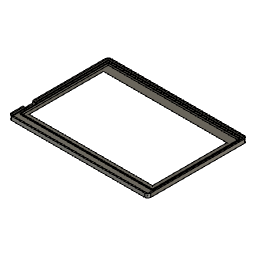
Soldered Inkplate 7 v1.0.0. Top v1.0.0. (Autodesk Fusion 360 design; units mm, degrees)
Autodesk Fusion 360 part; units mm, degrees
sketch "Sketch1" plane through (0, 0, 0) normal (0, 0, 1) x (1, 0, 0)
  line L0 (88.6, 66.25) -> (-88.6, 66.25)
  line L1 (-92.6, 62.25) -> (-92.6, -62.25)
  line L2 (-88.6, -66.25) -> (88.6, -66.25)
  line L3 (92.6, -62.25) -> (92.6, 62.25)
  line L4 (92.6, 66.25) -> (-92.6, -66.25) construction
  line L5 (-92.6, 66.25) -> (92.6, -66.25) construction
  line L6 (82.1, 49.46) -> (-82.1, 49.46)
  line L7 (-82.1, 49.46) -> (-82.1, -49.46)
  line L8 (-82.1, -49.46) -> (82.1, -49.46)
  line L9 (82.1, -49.46) -> (82.1, 49.46)
  line L10 (82.1, 49.46) -> (-82.1, -49.46) construction
  line L11 (-82.1, 49.46) -> (82.1, -49.46) construction
  arc A0 (-88.6, 66.25) -> (-92.6, 62.25) centre (-88.6, 62.25) ccw
  arc A1 (-92.6, -62.25) -> (-88.6, -66.25) centre (-88.6, -62.25) ccw
  arc A2 (88.6, -66.25) -> (92.6, -62.25) centre (88.6, -62.25) ccw
  arc A3 (92.6, 62.25) -> (88.6, 66.25) centre (88.6, 62.25) ccw
  dimension "d1" = 185.2
  dimension "d2" = 132.5
  dimension "d3" = 98.92
  dimension "d4" = 164.2
  dimension "d9" = 4
  constraint horizontal L0
  constraint perpendicular L0 L1
  constraint parallel L0 L2
  constraint parallel L1 L3
  constraint coincident L4 origin
  constraint coincident L5 origin
  constraint horizontal L6
  constraint perpendicular L6 L7
  constraint parallel L6 L8
  constraint parallel L7 L9
  constraint coincident L10 origin
  constraint coincident L11 origin
  constraint coincident L5.start L0
  constraint coincident L5.start L1
  constraint tangent L0 A0
  constraint tangent L1 A0
  constraint coincident L4.end L2
  constraint coincident L4.end L1
  constraint tangent L2 A1
  constraint tangent L1 A1
  constraint equal A0 A1
  constraint coincident L5.end L3
  constraint coincident L5.end L2
  constraint tangent L3 A2
  constraint tangent L2 A2
  constraint equal A0 A2
  constraint coincident L4.start L0
  constraint coincident L4.start L3
  constraint tangent L0 A3
  constraint tangent L3 A3
  constraint equal A0 A3
  measures "d1" distance of L4.end L5.end
  measures "d2" distance of L5.start L4.end
  measures "d3" distance of L6.end L7.end
  measures "d4" distance of L6.start L6.end
  measures "d9" radius of A0
extrude "Extrude1" add sketch "Sketch1" along normal blind 5
sketch "Sketch2" plane through (0, 0, 5) normal (0, 0, 1) x (-1, 0, 0)
  line L0 (-82.1, -49.46) -> (-82.1, 49.46)
  line L1 (-82.1, 49.46) -> (82.1, 49.46)
  line L2 (82.1, 49.46) -> (82.1, -49.46)
  line L3 (82.1, -49.46) -> (-82.1, -49.46)
  line L4 (-92.6, 62.25) -> (-92.6, -62.25)
  line L5 (-88.6, -66.25) -> (88.6, -66.25)
  line L6 (92.6, -62.25) -> (92.6, 62.25)
  line L7 (88.6, 66.25) -> (-88.6, 66.25)
  line L8 (-91.1, -64.75) -> (91.1, -64.75)
  line L9 (91.1, -64.75) -> (91.1, 64.75)
  line L10 (91.1, 64.75) -> (-91.1, 64.75)
  line L11 (-91.1, 64.75) -> (-91.1, -64.75)
  line L12 (-91.1, -64.75) -> (91.1, 64.75) construction
  line L13 (91.1, -64.75) -> (-91.1, 64.75) construction
  arc A0 (-92.6, -62.25) -> (-88.6, -66.25) centre (-88.6, -62.25) ccw
  arc A1 (88.6, -66.25) -> (92.6, -62.25) centre (88.6, -62.25) ccw
  arc A2 (92.6, 62.25) -> (88.6, 66.25) centre (88.6, 62.25) ccw
  arc A3 (-88.6, 66.25) -> (-92.6, 62.25) centre (-88.6, 62.25) ccw
  dimension "d7" = 1.5
  dimension "d8" = 1.5
  constraint horizontal L8
  constraint perpendicular L8 L9
  constraint parallel L8 L10
  constraint parallel L9 L11
  constraint coincident L12 origin
  constraint coincident L13 origin
  measures "d7" distance of L5 L8
  measures "d8" distance of L4 L11
extrude "Extrude2" cut sketch "Sketch2" against normal blind 3.1 contours L8 L9 L10 L11
chamfer "Chamfer1" distance 1.9 angle 45 4 edges at (-82.1, 0, 0) (0, -49.46, 0) (0, 49.46, 0) (82.1, 0, 0)
sketch "Sketch3" plane through (0, 0, 1.9) normal (0, 0, 1) x (-1, 0, 0)
  line L0 (82.1, 49.46) -> (82.1, -49.46)
  line L1 (82.1, -49.46) -> (-82.1, -49.46)
  line L2 (-82.1, -49.46) -> (-82.1, 49.46)
  line L3 (-82.1, 49.46) -> (82.1, 49.46)
  line L4 (-91.1, 64.75) -> (-91.1, -64.75)
  line L5 (-91.1, -64.75) -> (91.1, -64.75)
  line L6 (91.1, -64.75) -> (91.1, 64.75)
  line L7 (91.1, 64.75) -> (-91.1, 64.75)
  line L8 (0, 0) -> (0, -20) construction
  line L9 (-88.1, -61.75) -> (88.1, -61.75)
  line L10 (88.1, -61.75) -> (88.1, 55.45)
  line L11 (88.1, 55.45) -> (-88.1, 55.45)
  line L12 (-88.1, 55.45) -> (-88.1, -61.75)
  line L13 (-88.1, -61.75) -> (88.1, 55.45) construction
  line L14 (88.1, -61.75) -> (-88.1, 55.45) construction
  line L15 (-86.1, -59.75) -> (86.1, -59.75)
  line L16 (86.1, -59.75) -> (86.1, 53.45)
  line L17 (86.1, 53.45) -> (-86.1, 53.45)
  line L18 (-86.1, 53.45) -> (-86.1, -59.75)
  line L19 (-86.1, -59.75) -> (86.1, 53.45) construction
  line L20 (86.1, -59.75) -> (-86.1, 53.45) construction
  point P0 (0, -3.15)
  point P1 (0, -3.15)
  point P2 (0, -3.15)
  dimension "d19" = 3.15
  dimension "d20" = 3
  dimension "d21" = 3
  dimension "d22" = 2
  dimension "d23" = 2
  constraint coincident L8.start origin
  constraint vertical L8
  constraint coincident P2 L8
  constraint horizontal L9
  constraint perpendicular L9 L10
  constraint parallel L9 L11
  constraint parallel L10 L12
  constraint coincident L13 P2
  constraint coincident L14 P2
  constraint coincident P2 P1
  constraint horizontal L15
  constraint perpendicular L15 L16
  constraint parallel L15 L17
  constraint parallel L16 L18
  constraint coincident L19 P2
  constraint coincident L20 P2
  measures "d19" distance of L8.start P2
  measures "d20" distance of L5 L9
  measures "d21" distance of L4 L12
  measures "d22" distance of L9 L15
  measures "d23" distance of L12 L18
extrude "Extrude3" add sketch "Sketch3" along normal blind 1.2 contours L9 L10 L11 L12
chamfer "Chamfer2" distance 1.2 angle 45 4 edges at (0, 59.75, 3.1) (-86.1, 3.15, 3.1) (86.1, 3.15, 3.1) (0, -53.45, 3.1)
sketch "Sketch4" plane through (0, 0, 1.9) normal (0, 0, 1) x (-1, 0, 0)
  line L0 (-91.1, 64.75) -> (-91.1, -64.75)
  line L1 (-91.1, -64.75) -> (91.1, -64.75)
  line L2 (91.1, -64.75) -> (91.1, 64.75)
  line L3 (91.1, 64.75) -> (-91.1, 64.75)
  line L4 (-88.1, 55.45) -> (88.1, 55.45)
  line L5 (88.1, 55.45) -> (88.1, -61.75)
  line L6 (88.1, -61.75) -> (-88.1, -61.75)
  line L7 (-88.1, -61.75) -> (-88.1, 55.45)
  line L8 (88.1, 31.95) -> (91.1, 31.95)
  line L9 (91.1, 31.95) -> (91.1, 33.95)
  line L10 (91.1, 33.95) -> (88.1, 33.95)
  line L11 (88.1, 33.95) -> (88.1, 31.95)
  line L12 (89.1, 38.9967) -> (89.1, 53.7443) construction
  line L13 (92.6, -62.25) -> (92.6, 62.25)
  line L14 (89.1, 46.95) -> (88.1, 46.95)
  line L15 (88.1, 46.95) -> (88.1, 48.95)
  line L16 (88.1, 48.95) -> (89.1, 48.95)
  line L17 (89.1, 48.95) -> (89.1, 46.95)
  line L18 (88.6, 66.25) -> (-88.6, 66.25)
  dimension "d27" = 3.5
  dimension "d28" = 2
  dimension "d30" = 13
  dimension "d31" = 2
  dimension "d37" = 19.3
  constraint horizontal L8
  constraint vertical L9
  constraint horizontal L10
  constraint vertical L11
  constraint coincident L2 L9.end
  constraint coincident L5 L8.start
  constraint vertical L12
  constraint horizontal L14
  constraint vertical L15
  constraint horizontal L16
  constraint vertical L17
  constraint coincident L5 L15.end
  constraint coincident L12 L14.start
  measures "d27" distance of L12 L13
  measures "d28" distance of L14.start L16.end
  measures "d30" distance of L10 L14.start
  measures "d31" distance of L8.end L9.end
  measures "d37" vertical distance of L14.start L18.start
extrude "Extrude4" add sketch "Sketch4" along normal blind 3.1 contours L2 L5 L8 L9 L10 L11 | L5 L14 L15 L16 L17
sketch "Sketch5" plane through (-92.6, 0, 0) normal (-1, 0, 0) x (0, -1, 0)
  line L0 (-62.25, 0) -> (62.25, 0)
  line L1 (62.25, 0) -> (62.25, 5)
  line L2 (62.25, 5) -> (-62.25, 5)
  line L3 (-62.25, 5) -> (-62.25, 0)
  line L4 (46.95, 5) -> (33.95, 5)
  line L5 (33.95, 5) -> (33.95, 2)
  line L6 (33.95, 2) -> (46.95, 2)
  line L7 (46.95, 2) -> (46.95, 5)
  point P0 (66.25, 5)
  dimension "d34" = 13
  dimension "d35" = 3
  dimension "d36" = 19.3
  constraint horizontal L4
  constraint vertical L5
  constraint horizontal L6
  constraint vertical L7
  constraint coincident L2 L4.start
  measures "d34" distance of L4.start L4.end
  measures "d35" distance of L4.start L6.end
  measures "d36" distance of L4.start P0
extrude "Extrude5" cut sketch "Sketch5" against normal blind 2 contours L2 L4 L5 L6 L7
fillet "Fillet1" radius 2 4 edges at (-88.6, -46.95, 1.9) (-91.85, -46.95, 2) (-89.6, -33.95, 1.9) (-91.85, -33.95, 2)
fillet "Fillet2" radius 1 3 edges at (-88.1, -46.0454, 2.2267) (-88.1, -40.45, 1.9) (-88.1, -34.8546, 2.2267)
sketch "Sketch6" plane through (0, 0, 5) normal (0, 0, 1) x (-1, 0, 0)
  line L0 (91.1, 46.95) -> (92.6, 46.95)
  line L1 (92.6, 46.95) -> (92.6, 62.25)
  arc A0 (92.6, 62.25) -> (88.6, 66.25) centre (88.6, 62.25) ccw
  line L2 (88.6, 66.25) -> (-88.6, 66.25)
  arc A1 (-88.6, 66.25) -> (-92.6, 62.25) centre (-88.6, 62.25) ccw
  line L3 (-92.6, 62.25) -> (-92.6, -62.25)
  arc A2 (-92.6, -62.25) -> (-88.6, -66.25) centre (-88.6, -62.25) ccw
  line L4 (-88.6, -66.25) -> (88.6, -66.25)
  arc A3 (88.6, -66.25) -> (92.6, -62.25) centre (88.6, -62.25) ccw
  line L5 (92.6, -62.25) -> (92.6, 33.95)
  line L6 (92.6, 33.95) -> (88.1, 33.95)
  line L7 (88.1, 33.95) -> (88.1, 31.95)
  line L8 (88.1, 31.95) -> (91.1, 31.95)
  line L9 (91.1, 31.95) -> (91.1, -64.75)
  line L10 (91.1, -64.75) -> (-91.1, -64.75)
  line L11 (-91.1, -64.75) -> (-91.1, 64.75)
  line L12 (-91.1, 64.75) -> (91.1, 64.75)
  line L13 (91.1, 64.75) -> (91.1, 46.95)
  line L14 (91.1, -64.75) -> (-91.1, -64.75)
  line L15 (-91.1, -64.75) -> (-91.1, 64.75)
  line L16 (-91.1, 64.75) -> (91.1, 64.75)
  line L17 (91.1, 64.75) -> (91.1, -64.75)
  line L18 (91.1, -64.75) -> (-91.1, 64.75) construction
  line L19 (-91.1, -64.75) -> (91.1, 64.75) construction
  line L20 (90.1, -63.75) -> (-90.1, -63.75)
  line L21 (-90.1, -63.75) -> (-90.1, 63.75)
  line L22 (-90.1, 63.75) -> (90.1, 63.75)
  line L23 (90.1, 63.75) -> (90.1, -63.75)
  line L24 (90.1, -63.75) -> (-90.1, 63.75) construction
  line L25 (-90.1, -63.75) -> (90.1, 63.75) construction
  line L26 (91.1, 46.95) -> (90.1, 46.95)
  dimension "d44" = 1
  dimension "d45" = 1
  constraint horizontal L14
  constraint perpendicular L14 L15
  constraint parallel L14 L16
  constraint parallel L15 L17
  constraint coincident L18 origin
  constraint coincident L19 origin
  constraint coincident L9.end L10.start
  constraint horizontal L20
  constraint perpendicular L20 L21
  constraint parallel L20 L22
  constraint parallel L21 L23
  constraint coincident L24 origin
  constraint coincident L25 origin
  constraint coincident L0.start L13.end
  constraint coincident L23 L26.end
  constraint perpendicular L23 L26
  measures "d44" distance of L14 L20
  measures "d45" distance of L17 L23
extrude "Extrude6" add sketch "Sketch6" against normal blind 2 contours L8 L9 L10 L11 L12 L13 L14 L15 L16 L17 L20 L21 L22 L23 L26
chamfer "Chamfer3" distance 1 angle 45 10 edges at (-90.1, -55.35, 3) (-90.1, -55.35, 5) (-90.1, 15.9, 5) (-90.1, 15.9, 3) (0, -63.75, 5) (0, -63.75, 3) (90.1, 0, 5) (90.1, 0, 3) (0, 63.75, 5) (0, 63.75, 3)
equation "d10 = -2.90 mm - 0.2 mm"
